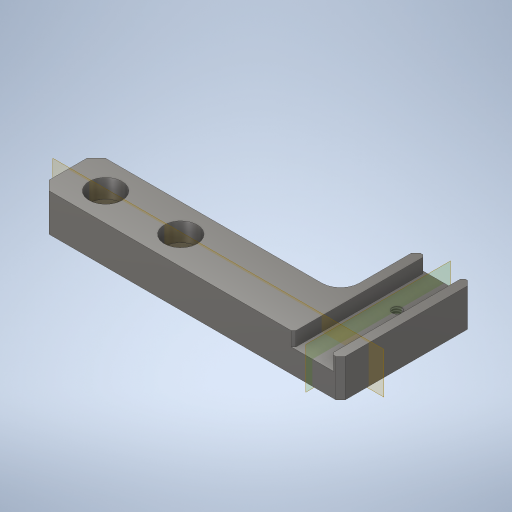
# Autodesk Inventor part: Holder - headbars - L - RH
Saved by Autodesk Inventor 2023 (Build 270158000, 158)
## iProperties
Created: 2019-01-08
Part Number: Holder - headbars - L - RH
Material: Stainless Steel
Document SubType Name: Modeling
Designer: Tanya
Density: 8 g/cm^3
Appearance: Semi-Polished
Author: Tanya
Autodesk Inventor part; units mm, degrees
ref_plane "YZ Plane" through (0, 0, 0) normal (1, 0, 0) x (0, 1, 0)
ref_plane "XZ Plane" through (0, 0, 0) normal (0, 1, 0) x (-1, 0, 0)
ref_plane "XY Plane" through (0, 0, 0) normal (0, 0, 1) x (1, 0, 0)
sketch "Sketch1" plane through (0, 0, 0) normal (0, 1, 0) x (-1, 0, 0)
  line L0 (0, -85.725) -> (0, 14.2875) projected
  line L1 (-90.17, 0) -> (52.07, 0) projected
  line L2 (-50.8, -52.3875) -> (31.75, -52.3875)
  line L3 (-69.85, -71.4375) -> (31.75, -71.4375)
  line L4 (-69.85, -26.9875) -> (-50.8, -26.9875)
  line L5 (-50.8, -26.9875) -> (-50.8, -52.3875)
  line L6 (-69.85, -26.9875) -> (-69.85, -71.4375)
  line L7 (-53.975, -26.9875) -> (-66.675, -26.9875) construction
  line L8 (-66.675, -26.9875) -> (-66.675, -71.4375) construction
  line L9 (-66.675, -71.4375) -> (-53.975, -71.4375) construction
  line L10 (-53.975, -71.4375) -> (-53.975, -26.9875) construction
  line L11 (-60.325, -26.9875) -> (-60.325, -71.4375) construction
  line L12 (31.75, -52.3875) -> (31.75, -71.4375)
  point P0 (0, 0)
  dimension "d3" = 26.9875
  dimension "d5" = 19.05
  dimension "d6" = 3.175
  dimension "d7" = 50.8
  dimension "d11" = 19.05
  dimension "d57" = 101.6
  dimension "d58" = 12.7
  dimension "d59" = 44.45
  constraints: 22 end point, 2 midpoint, 2 parallel, 2 perpendicular, 2 point on line, 1 horizontal
  measures "d3" distance between parallel lines of L1 L4
  measures "d5" distance between parallel lines of L6 L5
  measures "d6" distance between parallel lines of L6 L8
  measures "d7" distance between parallel lines of L0 L5
  measures "d11" distance between parallel lines of L3 L2
  measures "d57" distance between parallel lines of L6 L12
  measures "d58" distance between parallel lines of L8 L10
  measures "d59" distance between parallel lines of L7 L3
extrude "Extrusion1" add sketch "Sketch1" along normal mid plane 12.7
sketch "Sketch2" plane through (0, 6.35, 0) normal (0, 1, 0) x (1, 0, 0)
  line L0 (-31.75, 52.3875) -> (50.8, 52.3875) projected
  line L1 (50.8, 52.3875) -> (50.8, 26.9875) projected
  line L2 (50.8, 26.9875) -> (69.85, 26.9875) projected
  line L3 (69.85, 26.9875) -> (69.85, 71.4375) projected
  line L4 (69.85, 71.4375) -> (-31.75, 71.4375) projected
  line L5 (50.8, 26.9875) -> (69.85, 26.9875) projected
  line L6 (69.85, 71.4375) -> (-31.75, 71.4375) projected
  line L7 (53.975, 26.9875) -> (66.675, 26.9875)
  line L8 (66.675, 26.9875) -> (66.675, 71.4375)
  line L9 (66.675, 71.4375) -> (53.975, 71.4375)
  line L10 (53.975, 71.4375) -> (53.975, 26.9875)
  line L11 (60.325, -63.5) -> (60.325, 99.2856) construction
  line L12 (102.235, 0) -> (-124.46, 0) projected
  line L13 (-31.75, 71.4375) -> (-31.75, 52.3875) projected
  point P0 (0, 0)
  point P1 (60.325, 26.9875)
  dimension "d60" = 12.7
  dimension "d61" = 6.35
  constraints: 10 end point, 3 point on line, 2 parallel, 1 horizontal, 1 midpoint, 1 perpendicular
  measures "d60" distance between parallel lines of L8 L10
  measures "d61" distance between parallel lines of L11 L10
extrude "Extrusion2" cut sketch "Sketch2" against normal blind 4.7625 contours L4 L8 L2 L10
chamfer "Chamfer1" distance 1.5875 angle 45 3 edges at (69.85, 0, -26.9875) (69.85, 0, -71.4375) (50.8, 0, -26.9875)
sketch "Sketch4" plane through (0, 1.5875, 0) normal (0, 1, 0) x (1, 0, 0)
  line L0 (53.975, 71.4375) -> (66.675, 71.4375) projected
  line L1 (53.975, 26.9875) -> (53.975, 71.4375) projected
  line L2 (66.675, 26.9875) -> (53.975, 26.9875) projected
  line L3 (66.675, 71.4375) -> (66.675, 26.9875) projected
  point P0 (0, 0)
  point P1 (60.325, 42.8625)
  dimension "d44" = 15.875
  dimension "d46" = 6.35
  measures "d44" distance from line of point (60.325, 42.862) L2
  measures "d46" distance from line of point (60.325, 42.862) L3
hole "Hole2" at (60.325, 1.5875, -42.8625) direction (0, -1, 0) diameter 3.302 end through all thread size "8-32 UNC" class "2B" standard "ANSI Unified Screw Threads"
chamfer "Chamfer3" distance 0.7937 angle 45 4 edges at (53.975, 3.9687, -26.9875) (66.675, 3.9687, -26.9875) (53.975, 3.9687, -71.4375) (66.675, 3.9687, -71.4375)
sketch "Sketch5" plane through (0, 6.35, 0) normal (0, 1, 0) x (1, 0, 0)
  line L0 (53.1813, 71.4375) -> (53.975, 70.6437) projected
  line L1 (53.1813, 71.4375) -> (-31.75, 71.4375) projected
  line L2 (-31.75, 71.4375) -> (-31.75, 52.3875) projected
  line L3 (-31.75, 52.3875) -> (50.8, 52.3875) projected
  line L4 (50.8, 52.3875) -> (50.8, 28.575) projected
  line L5 (52.3875, 26.9875) -> (50.8, 28.575) projected
  line L6 (52.3875, 26.9875) -> (53.1813, 26.9875) projected
  line L7 (53.975, 27.7812) -> (53.1813, 26.9875) projected
  line L8 (53.975, 27.7812) -> (53.975, 70.6437) projected
  line L9 (-31.75, 71.4375) -> (-31.75, 52.3875) construction
  line L10 (-31.75, 61.9125) -> (53.975, 61.9125) construction
  point P0 (0, 0)
  point P1 (-19.05, 61.9125)
  point P2 (6.35, 61.9125)
  dimension "d62" = 12.7
  dimension "d63" = 25.4
  constraints: 3 point on line, 2 end point, 1 horizontal, 1 midpoint
  measures "d62" distance from line of point (-19.05, 61.912) L2
  measures "d63" distance of point (6.35, 61.912) point (-19.05, 61.912)
hole "Hole3" at (-19.05, 6.35, -61.9125) at (6.35, 6.35, -61.9125) direction (0, -1, 0) diameter 6.7564 end through all counterbore diameter 11.1252 counterbore depth 6.35 clearance for "Socket Head Cap Screw" size "1/4" standard "Ansi Unified Screw Threads"
chamfer "Chamfer4" distance 3.175 angle 45 2 edges at (-31.75, 0, -52.3875) (-31.75, 0, -71.4375)
fillet "Fillet2" radius 6.35 1 edges at (50.8, 0, -52.3875)
mirror "Mirror1" about plane through (0, 0, 0) normal (0, 0, 1) remove original yes
ref_plane "Work Plane3" through (-28.575, -6.35, 61.9125) normal (0, 0, 1) x (1, 0, 0)
ref_plane "Work Plane4" through (60.325, -6.35, 46.0375) normal (-1, 0, 0) x (0, 0, 1)
equation "\"d3\" = 0.5 * d2"
equation "\"d7\" = 0.5 * d4"
equation "\"d11\" = d10"
equation "\"d61\" = 0.5 * d60"
equation "\"d2\" = 53.975"
equation "\"d4\" = 101.6"
equation "\"d10\" = 19.05"
body "Solid1"
